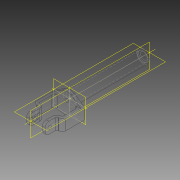
# Autodesk Inventor part: Fork_Example
Saved by Autodesk Inventor 2015 (Build 190159000, 159)
## iProperties
Created: 2015-01-16
Part Number: Fork_Example
Material: Generic
Document SubType Name: Modeling
Designer: admin
Density: 1 g/cm^3
Appearance: Default
Author: admin
Autodesk Inventor part; units mm, degrees
sketch "Sketch1" plane through (0, 0, 0) normal (0, 1, 0) x (-1, 0, 0)
  line L0 (19.6, 0) -> (-19.6, 0) projected
  line L1 (0, -19.6) -> (0, 19.6) projected
  circle A0 centre (0, 0) radius 14
  dimension "d0" = 28
  constraints: 1 centre point, 1 coincident
  measures "d0" diameter of A0
extrude "Extrusion1" add sketch "Sketch1" along normal blind 165
chamfer "Chamfer1" distance 2 angle 45 1 edges at (14, 165, 0)
shell "Shell1" thickness 3 removed faces 1 at (-2.994, 165, 1.0653)
sketch "Sketch2" plane through (0, 0, 0) normal (0, -1, 0) x (1, 0, 0)
  circle A0 centre (0, 0) radius 14 projected
  circle A1 centre (0, 0) radius 11 projected
  arc A2 (9.9692, 14.9871) -> (-9.9692, 14.9871) centre (0, 0) ccw
  line L0 (0, 0) -> (32.5, 0)
  line L1 (32.5, 0) -> (32.5, -25)
  line L2 (32.5, 0) -> (9.9692, 14.9871)
  line L3 (32.5, -25) -> (0, -30)
  line L4 (0, 0) -> (0, -51.2794) construction
  line L5 (-32.5, 0) -> (-32.5, -25)
  line L6 (-32.5, 0) -> (-9.9692, 14.9871)
  line L7 (-32.5, -25) -> (0, -30)
  dimension "d7" = 36
  dimension "d8" = 32.5
  dimension "d9" = 25
  dimension "d10" = 30
  dimension "d11" = 32.5
  constraints: 16 end point, 3 symmetric about line, 2 point on circle, 1 centre point, 1 coincident, 1 horizontal, 1 horizontal alignment, 1 perpendicular, 1 tangent, 1 vertical
  measures "d7" diameter of A2
  measures "d8" distance of L0.start L0.end
  measures "d9" distance of L0.end L1.end
  measures "d10" distance of L3.end A0.centre
  measures "d11" horizontal distance of L1.end L3.end
extrude "Extrusion2" add sketch "Sketch2" along normal blind 7 contours A0 | A1 | L2 L1 L3 L7 L5 L6 A2
ref_plane "Work Plane1" through (0, 0, -14) normal (0, 0, 1) x (1, 0, 0)
sketch "Sketch3" plane through (0, -7, 0) normal (0, -1, 0) x (1, 0, 0)
  line L0 (32.5, -25) -> (32.5, 0) projected
  line L1 (32.5, 0) -> (9.9692, 14.9871) projected
  arc A0 (9.9692, 14.9871) -> (-9.9692, 14.9871) centre (0, 0) ccw projected
  line L2 (-9.9692, 14.9871) -> (-32.5, 0) projected
  line L3 (-32.5, 0) -> (-32.5, -25) projected
  line L4 (-32.5, -25) -> (0, -30) projected
  line L5 (0, -30) -> (32.5, -25) projected
  line L6 (32.5, 0) -> (26.5, 0)
  line L7 (26.5, 0) -> (26.5, -25)
  line L8 (26.5, -25) -> (32.5, -25)
  line L9 (32.5, -25) -> (32.5, 0)
  dimension "d14" = 6
  constraints: 8 end point, 2 parallel, 1 horizontal, 1 perpendicular
  measures "d14" distance of L7.end L8.end
sketch "Sketch4" plane through (0, 0, -14) normal (0, 0, 1) x (1, 0, 0)
  line L0 (32.5, 0) -> (32.5, -7) projected
  line L1 (32.5, -7) -> (32.5, -41.5)
  line L2 (25, -49) -> (24, -49)
  line L3 (20.5, -52.5) -> (20.5, -75)
  arc A0 (25, -49) -> (32.5, -41.5) centre (25, -41.5) ccw
  arc A1 (24, -49) -> (20.5, -52.5) centre (24, -52.5) ccw
  point P0 (0, 0)
  point P1 (32.5, -49)
  point P2 (20.5, -49)
  dimension "d16" = 42
  dimension "d17" = 12
  dimension "d18" = 26
  dimension "d19" = 7.5
  dimension "d20" = 3.5
  constraints: 6 end point, 4 point on circle, 4 point on line, 4 tangent, 2 centre point, 2 vertical, 1 horizontal
  measures "d16" distance of L0.end point (32.5, -49)
  measures "d17" distance of point (32.5, -49) point (20.5, -49)
  measures "d18" distance of point (20.5, -49) L3.end
  measures "d19" radius of A0
  measures "d20" radius of A1
sweep "Sweep1" add profiles "Sketch3" path "Sketch4" contours L8 L7 L6 L0
fillet "Fillet1" radius 6 1 edges at (26.5, -7, -12.5)
fillet "Fillet2" radius 8 2 edges at (17.5, -75, -25) (17.5, -75, 0)
ref_plane "Work Plane2" through (12, -52.5, -25) normal (-1, 0, 0) x (0, 0, 1)
sketch "Sketch5" plane through (12, -52.5, -25) normal (-1, 0, 0) x (0, 0, 1)
  arc A0 (17, -22.5) -> (25, -14.5) centre (17, -14.5) ccw projected
  line L0 (25, 0) -> (25, -14.5) projected
  line L1 (25, 0) -> (0, 0) projected
  line L2 (0, 0) -> (0, -14.5) projected
  arc A1 (0, -14.5) -> (8, -22.5) centre (8, -14.5) ccw projected
  line L3 (17, -22.5) -> (8, -22.5) projected
  circle A2 centre (12.5, -12.5) radius 4
  line L4 (7.5, -7.5) -> (17.5, -7.5)
  line L5 (17.5, -7.5) -> (17.5, -17.5)
  line L6 (17.5, -17.5) -> (7.5, -17.5)
  line L7 (7.5, -17.5) -> (7.5, -7.5)
  point P0 (25, 52.5)
  point P1 (17.5, -12.5)
  point P2 (12.5, -22.5)
  point P3 (12.5, -17.5)
  dimension "d26" = 8
  dimension "d27" = 10
  dimension "d28" = 10
  dimension "d29" = 10
  constraints: 8 end point, 3 midpoint, 2 parallel, 2 vertical alignment, 1 centre point, 1 horizontal, 1 horizontal alignment, 1 perpendicular
  measures "d26" diameter of A2
  measures "d27" distance from line of L3 A2.centre
  measures "d28" distance of L4.end L5.end
  measures "d29" distance of L4.start L4.end
sketch "Sketch6" plane through (14.5, -52.5, -25) normal (-1, 0, 0) x (0, 0, 1)
  arc A0 (17, -22.5) -> (25, -14.5) centre (17, -14.5) ccw projected
  line L0 (8, -22.5) -> (17, -22.5) projected
  arc A1 (0, -14.5) -> (8, -22.5) centre (8, -14.5) ccw projected
  line L1 (0, 0) -> (0, -14.5) projected
  line L2 (0, 0) -> (25, 0) projected
  line L3 (25, 0) -> (25, -14.5) projected
  line L4 (7.5, -0.5) -> (17.5, -0.5)
  line L5 (17.5, -0.5) -> (17.5, -20.5)
  line L6 (17.5, -20.5) -> (7.5, -20.5)
  line L7 (7.5, -20.5) -> (7.5, -0.5)
  point P0 (25, 52.5)
  point P1 (12.5, -20.5)
  point P2 (12.5, -22.5)
  dimension "d30" = 10
  dimension "d31" = 20
  dimension "d32" = 2
  constraints: 8 end point, 2 midpoint, 2 parallel, 1 horizontal, 1 perpendicular, 1 vertical alignment
  measures "d30" distance of L4.start L4.end
  measures "d31" distance of L4.end L5.end
  measures "d32" distance of point (12.5, -22.5) point (12.5, -20.5)
loft "Loft1" add profiles "Sketch6", "Sketch5" contours L4 L5 L6 L7 / A2 | L4 L5 L6 L7
extrude "Extrusion3" cut sketch "Sketch5" against normal up to next contours A2
mirror "Mirror1" about plane through (0, 0, 0) normal (1, 0, 0) of "Fillet2", "Sweep1", "Loft1", "Extrusion3", "Fillet1"
sketch "Sketch7" plane through (0, -7, 0) normal (0, -1, 0) x (1, 0, 0)
  line L0 (-20.5, -25) -> (-32.5, -25) projected
  line L1 (-32.5, -25) -> (0, -30) projected
  line L2 (0, -30) -> (32.5, -25) projected
  line L3 (32.5, -25) -> (20.5, -25) projected
  line L4 (20.5, 0) -> (20.5, -25) projected
  line L5 (20.5, 0) -> (32.5, 0) projected
  line L6 (32.5, 0) -> (9.9692, 14.9871) projected
  arc A0 (9.9692, 14.9871) -> (-9.9692, 14.9871) centre (0, 0) ccw projected
  line L7 (-9.9692, 14.9871) -> (-32.5, 0) projected
  line L8 (-32.5, 0) -> (-20.5, 0) projected
  line L9 (-20.5, -25) -> (-20.5, 0) projected
hole "Hole1" at (0, -7, 0) direction (0, 1, 0) diameter 8 end through all
chamfer "Chamfer2" distance 2 angle 45 2 edges at (16.25, 0, -27.5) (-32.5, 0, -12.5)
body "Solid1"
